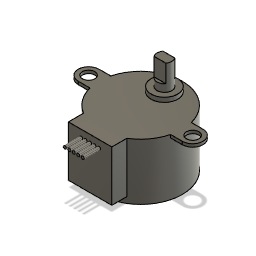
28BYJ_48_5V_Stepper Motor (Autodesk Fusion 360 design; units mm, degrees)
Autodesk Fusion 360 part; units mm, degrees
sketch "Skizze1" plane through (0, 0, 0) normal (0, 1, 0) x (1, 0, 0)
  circle A0 centre (0, 0) radius 14
  circle A1 centre (17.5, 0) radius 2.1
  circle A2 centre (-17.5, 0) radius 2.1
  circle A3 centre (0, 8) radius 4.5
  circle A4 centre (0, 8) radius 2.5
  line L0 (2, 9.5) -> (-2, 9.5)
  line L1 (-2, 6.5) -> (2, 6.5)
  line L2 (0, 0) -> (0, 14) construction
  line L3 (0, 0) -> (0, -17) construction
  line L4 (0, -17) -> (7.3, -17)
  line L5 (0, -17) -> (-7.3, -17)
  line L6 (-7.3, -17) -> (-7.3, -11.9461)
  line L7 (7.3, -17) -> (7.3, -11.9461)
  line L8 (0, 0) -> (-17.5, 0) construction
  line L9 (0, 0) -> (17.5, 0) construction
  line L10 (17.5, 0) -> (17.5, 3.5) construction
  line L11 (17.5, 0) -> (17.5, -3.5) construction
  line L12 (17.5, 3.5) -> (13.5554, 3.5)
  line L13 (-13.5554, 3.5) -> (-17.5, 3.5)
  arc A5 (-17.5, 3.5) -> (-17.5, -3.5) centre (-17.5, 0) ccw
  line L14 (17.5, -3.5) -> (13.5554, -3.5)
  line L15 (-13.5554, -3.5) -> (-17.5, -3.5)
  arc A6 (17.5, -3.5) -> (17.5, 3.5) centre (17.5, 0) ccw
  dimension "d1" = 28
  dimension "d2" = 4.2
  dimension "d3" = 4.2
  dimension "d4" = 17.5
  dimension "d5" = 17.5
  dimension "d6" = 9
  dimension "d7" = 8
  dimension "d8" = 5
  dimension "d9" = 3
  dimension "d10" = 17
  dimension "d11" = 7.3
  dimension "d12" = 7.3
  dimension "d13" = 7
  dimension "d14" = 7
  constraint coincident A0.centre L2.start
  constraint concentric A3 A4
  constraint coincident A4 L0.start
  constraint coincident A4 L0.end
  constraint horizontal L0
  constraint coincident A4 L1.start
  constraint coincident A4 L1.end
  constraint parallel L0 L1
  constraint equal L0 L1
  constraint coincident A0 L2.end
  constraint vertical L2
  constraint coincident A3.centre L2
  constraint parallel L2 L3
  constraint perpendicular L3 L4
  constraint perpendicular L3 L5
  constraint coincident A0 L6.end
  constraint perpendicular L5 L6
  constraint coincident A0 L7.end
  constraint perpendicular L4 L7
  constraint concentric A1 A6
  constraint concentric A2 A5
  constraint coincident A2.centre L8.end
  constraint perpendicular L2 L8
  constraint coincident A1.centre L9.end
  constraint perpendicular L3 L9
  constraint perpendicular L9 L10
  constraint tangent L12 A5
  constraint perpendicular L9 L11
  constraint tangent A5 L14
  constraint coincident A0 L13.start
  constraint collinear L12 L13
  constraint coincident A0 L15.start
  constraint collinear L14 L15
  constraint coincident A0 L12.end
  constraint coincident A0 L14.end
  measures "d1" diameter of A0
  measures "d2" diameter of A1
  measures "d3" diameter of A2
  measures "d4" distance of A0.centre A2.centre
  measures "d5" distance of A0.centre A1.centre
  measures "d6" diameter of A3
  measures "d7" distance of A0.centre A3.centre
  measures "d8" diameter of A4
  measures "d9" distance of L0 L1
  measures "d10" distance of A0.centre L3.end
  measures "d11" distance of L3.end L4.end
  measures "d12" distance of L3.end L5.end
  measures "d13" diameter of A6
  measures "d14" diameter of A5
extrude "Extrusion1" add sketch "Skizze1" against normal blind 19 contours A0 | A3 | A4 L0 L1 | A4 L0 | A4 L1
extrude "Extrusion2" add sketch "Skizze1" against normal blind 17 contours A0 L4 L5 L6 L7
extrude "Extrusion3" add sketch "Skizze1" against normal blind 1 contours A0 L12 L14 A6 | A0 L13 A5 L15
extrude "Extrusion4" add sketch "Skizze1" along normal blind 1.5 contours A3
extrude "Extrusion5" add sketch "Skizze1" along normal blind 10 contours A4 L0 L1
extrude "Extrusion6" add sketch "Skizze1" along normal blind 4 contours A4 L0 | A4 L1
sketch "Skizze2" plane through (0, 0, 17) normal (0, 0, 1) x (1, 0, 0)
  line L0 (7.3, 0) -> (-7.3, 0)
  line L1 (-7.3, 0) -> (-7.3, -17)
  line L2 (-7.3, -17) -> (7.3, -17)
  line L3 (7.3, -17) -> (7.3, 0)
  circle A0 centre (0, -2.5) radius 0.5
  circle A1 centre (-1.5, -2.5) radius 0.5
  circle A2 centre (-3, -2.5) radius 0.5
  circle A3 centre (1.5, -2.5) radius 0.5
  circle A4 centre (3, -2.5) radius 0.5
extrude "Extrusion7" add sketch "Skizze2" along normal blind 5.5 contours A0 | A1 | A2 | A3 | A4
equation "d25 = 10.00 mm - 6 mm"
